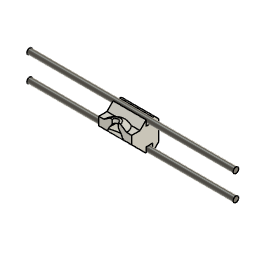
ForkHeightParts_FullAssembly_PESTA (Autodesk Fusion 360 archive; units mm, degrees)
design "AlinhadorEncoder"
Autodesk Fusion 360 part; units mm, degrees
sketch "Sketch1" plane through (0, 0, 0) normal (1, 0, 0) x (0, 1, 0) in component "Empilhador"
  circle A0 centre (0, 6.1) radius 1.35
  circle A1 centre (0, -6.1) radius 1.35
  line L0 (0, 4.75) -> (0, -4.75)
  dimension "d1" = 2.7
  dimension "d2" = 2.7
  dimension "d3" = 9.5
  constraint coincident A0 L0.start
  constraint coincident A1 L0.end
  constraint vertical L0
  constraint vertical origin L0.start
  constraint vertical A0.centre L0.start
  constraint vertical A1.centre L0.end
  constraint midpoint origin L0
  measures "d1" diameter of A0
  measures "d2" diameter of A1
  measures "d3" distance of L0.start L0.end
extrude "Extrude1" add sketch "Sketch1" along normal blind 50 and the other way blind 50 makes body 1 at (33.3333, -0.6364, 4.9094) makes body 2 at (33.3333, -0.694, -7.2579) in component "Empilhador"
sketch "Sketch1 (2)" plane through (0, 0, 0) normal (0, 1, 0) x (1, 0, 0) in component "Fundo"
  line L0 (8, -4.35) -> (-8, -4.35)
  line L1 (-8, -4.35) -> (-8, 4.35)
  line L2 (-8, 4.35) -> (8, 4.35)
  line L3 (8, 4.35) -> (8, -4.35)
  point P0 (0, -4.35)
  point P1 (8, 0)
  dimension "d8" = 8.7
  dimension "d9" = 16
  constraint horizontal L0
  constraint vertical L1
  constraint horizontal L2
  constraint vertical L3
  constraint midpoint L0 P0
  constraint midpoint L3 P1
  constraint vertical origin P0
  constraint horizontal origin P1
  measures "d8" distance of L0.start L2.end
  measures "d9" distance of L0.start L0.end
extrude "Extrude1'" add sketch "Sketch1 (2)" along normal blind 4 and the other way blind 1.5 separate body makes body 3 in component "Fundo"
sketch "Sketch2" plane through (0, -1.5, 0) normal (0, -1, 0) x (1, 0, 0) in component "Fundo"
  line L0 (-8, -4.35) -> (8, -4.35)
  line L1 (8, -4.35) -> (8, 4.35)
  line L2 (8, 4.35) -> (-8, 4.35)
  line L3 (-8, 4.35) -> (-8, -4.35)
  line L4 (-8, 7) -> (8, 7)
  line L5 (8, 7) -> (8, -7)
  line L6 (8, -7) -> (-8, -7)
  line L7 (-8, -7) -> (-8, 7)
  point P0 (0, 7)
  point P1 (-8, 0)
  dimension "d14" = 16
  dimension "d15" = 14
  constraint horizontal L4
  constraint vertical L5
  constraint horizontal L6
  constraint vertical L7
  constraint midpoint L4 P0
  constraint midpoint L7 P1
  constraint vertical origin P0
  constraint horizontal origin P1
  measures "d14" distance of L4.start L4.end
  measures "d15" distance of L4.start L6.end
extrude "Extrude2" add sketch "Sketch2" along normal blind 3 bodies 3 in component "Fundo"
chamfer "Chamfer1" distance 3 angle 45 2 edges at (0, -4.5, 7) (0, -4.5, -7) on bodies 3 in component "Fundo"
sketch "Sketch3" plane through (0, 0, 4.35) normal (0, 0, 1) x (-1, 0, 0) in component "Fundo"
  line L0 (-8, 1.5) -> (-8, -4)
  line L1 (-8, -4) -> (8, -4)
  line L2 (8, -4) -> (8, 1.5)
  line L3 (8, 1.5) -> (-8, 1.5)
  line L4 (-8, -1.6) -> (8, -1.6)
  line L5 (8, -1.6) -> (8, -4.6)
  line L6 (8, -4.6) -> (-8, -4.6)
  line L7 (-8, -4.6) -> (-8, -1.6)
  dimension "d19" = 3
  dimension "d22" = 3.1
  constraint horizontal L4
  constraint vertical L5
  constraint horizontal L6
  constraint vertical L7
  constraint coincident L2 L5.end
  measures "d19" distance of L4.start L6.end
  measures "d22" distance of L0.start L4.start
extrude "Extrude3" add sketch "Sketch3" along normal blind 2.25 and the other way blind 11.75 contours L0 L1 L2 L4 L5 L7 | L1 L5 L6 L7 bodies 3 in component "Fundo"
chamfer "Chamfer2" distance 2.2 angle 45 2 edges at (0, 4.6, -7.4) (0, 4.6, 6.6) on bodies 3 in component "Fundo"
sketch "Sketch5" plane through (0, -4.5, 0) normal (0, -1, 0) x (1, 0, 0) in component "Fundo"
  line L0 (-8, -4) -> (8, -4)
  line L1 (8, -4) -> (8, 4)
  line L2 (8, 4) -> (-8, 4)
  line L3 (-8, 4) -> (-8, -4)
  circle A0 centre (0, 0) radius 3.5
  dimension "d39" = 7
  constraint coincident A0.centre origin
  measures "d39" diameter of A0
extrude "Extrude7" cut sketch "Sketch5" against normal blind 12 contours A0 bodies 3 in component "Fundo"
extrude "Extrude8" add 1 faces at (-6.5, -4.5, 0) along direction (0, -1, 0) blind 4 on bodies 3 bodies 3 in component "Fundo"
sketch "Sketch6" plane through (0, 0, 4) normal (0, 0, 1) x (-1, 0, 0) in component "Fundo"
  line L0 (-8, 4.5) -> (8, 4.5)
  line L1 (8, 4.5) -> (8, 8.5)
  line L2 (8, 8.5) -> (-8, 8.5)
  line L3 (-8, 8.5) -> (-8, 4.5)
  circle A0 centre (0, 8.5) radius 1.5
  dimension "d44" = 3
  constraint midpoint L2 A0.centre
  measures "d44" diameter of A0
extrude "Extrude9" cut sketch "Sketch6" against normal blind 3.25 contours L2 A0 picked at (-0.3665, 8.1599) bodies 3 in component "Fundo"
fillet "Fillet2" radius 8.25 1 edges at (0, -7, 3.5) on bodies 3 in component "Fundo"
sketch "Sketch7" plane through (0, 0, 4) normal (0, 0, 1) x (-1, 0, 0) in component "Fundo"
  arc A0 (-1.5, 8.5) -> (1.5, 8.5) centre (0, 8.5) ccw
  line L0 (-1.5, 8.5) -> (-8, 8.5)
  line L1 (-8, 8.5) -> (-8, 4.5)
  line L2 (-8, 4.5) -> (8, 4.5)
  line L3 (8, 4.5) -> (8, 8.5)
  line L4 (8, 8.5) -> (1.5, 8.5)
  circle A1 centre (0, 8.5) radius 1.5
  circle A2 centre (0, 8.5) radius 2.5
  dimension "d49" = 5
  constraint concentric A0 A1
  constraint concentric A1 A2
  measures "d49" diameter of A2
extrude "Extrude10" add sketch "Sketch7" along normal blind 2 contours A0 L0 L4 A1 A2 bodies 3 in component "Fundo"
chamfer "Chamfer3" distance 3 distance2 2 1 edges at (0, -6, 4) measured on face at (-6.1296, -6.921, 4.0006) on bodies 3 in component "Fundo"
chamfer "Chamfer4" distance 4 angle 45 1 edges at (0, -8.5, -4) on bodies 3 in component "Fundo"
fillet "Fillet4" radius 1 1 edges at (0, -5, -3.5) on bodies 3 in component "Fundo"
component "Fundo" placed x (1, 0, 0) y (0, 1, 0) z (0, 0, 1) at (0, 0, 0)
component "Empilhador" placed x (1, 0, 0) y (0, 1, 0) z (0, 0, 1) at (0, 0, 0)
equation "d23 = 14 mm - 2.25 mm"
